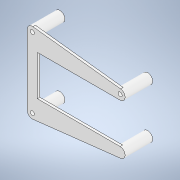
# Autodesk Inventor part: Support_LIDAR
Saved by Autodesk Inventor 2022 (Build 260153000, 153)
## iProperties
Created: 2021-07-03
Part Number: Support_LIDAR
Material: Générique
Document SubType Name: Modeling
Designer: utilisateur
Density: 1 g/cm^3
Appearance: Par défaut(1)
Author: utilisateur
Autodesk Inventor part; units mm, degrees
ref_plane "YZ Plane" through (0, 0, 0) normal (1, 0, 0) x (0, 1, 0)
ref_plane "XZ Plane" through (0, 0, 0) normal (0, 1, 0) x (-1, 0, 0)
ref_plane "XY Plane" through (0, 0, 0) normal (0, 0, 1) x (1, 0, 0)
sketch "Esquisse2" plane through (0, 0, 0) normal (0, 0, 1) x (1, 0, 0)
  circle A0 centre (42, 20) radius 1.65
  circle A1 centre (-28, 28) radius 1.65
  circle A2 centre (-28, -28) radius 1.65
  circle A3 centre (42, -20) radius 1.65 construction
  circle A4 centre (0, 0) radius 33 construction
  line L0 (-42, -20) -> (42, -20) construction
  line L1 (42, -20) -> (42, 20) construction
  line L2 (42, 20) -> (-42, 20) construction
  line L3 (-42, 20) -> (-42, -20) construction
  line L4 (-42, -20) -> (42, 20) construction
  line L5 (42, -20) -> (-42, 20) construction
  line L6 (28, -28) -> (-28, -28) construction
  line L7 (-28, -28) -> (-28, 28) construction
  line L8 (-28, 28) -> (28, 28) construction
  line L9 (28, 28) -> (28, -28) construction
  line L10 (28, -28) -> (-28, 28) construction
  line L11 (-28, -28) -> (28, 28) construction
  circle A5 centre (-28, 28) radius 4
  circle A6 centre (-28, -28) radius 4
  circle A7 centre (42, 20) radius 4
  circle A8 centre (42, -20) radius 4
  line L12 (-32, 28) -> (-32, -28)
  line L13 (46, 20) -> (46, -20)
  line L14 (38, 20) -> (38, -20)
  line L15 (-24, 28) -> (-24, -28)
  line L16 (-27.5458, 31.9741) -> (42.4542, 23.9741)
  line L17 (-27.5458, -31.9741) -> (42.4542, -23.9741)
  line L18 (42, -16) -> (-24, -16)
  line L19 (42, 16) -> (-24, 16)
  point P0 (14.25, 0)
  point P1 (38, 16)
  point P2 (38, -16)
  dimension "d4" = 56
  dimension "d5" = 56
  dimension "d6" = 40
  dimension "d7" = 84
  dimension "d8" = 3.3
  dimension "d9" = 66
  dimension "d10" = 8
  constraints: 40 end point, 14 point on circle, 9 centre point, 9 tangent, 8 point on line, 6 equal radius, 5 coincident, 4 midpoint, 4 parallel, 4 perpendicular, 2 horizontal, 1 vertical
  measures "d4" distance of L7.end L9.start
  measures "d5" distance of L9.start L9.end
  measures "d6" distance of L1.start L1.end
  measures "d7" distance of L1.end L3.start
  measures "d8" diameter of A0
  measures "d9" diameter of A4
  measures "d10" diameter of A7
extrude "Extrusion2" add sketch "Esquisse2" along normal blind 2 contours A5 | L15 A6 L12 A5 | A5 L16 A7 L14 L19 L15 | A7 | A6 | L18 L14 A8 L17 A6 L15 | L14 A7 L19 | L18 A8 L14 | A8
extrude "Extrusion3" add sketch "Esquisse2" against normal blind 20 contours A5 | A7 | A6 | A8
